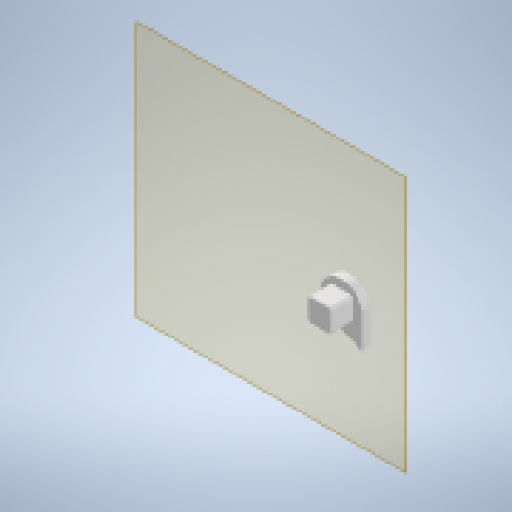
# Autodesk Inventor part: Arm
Saved by Autodesk Inventor 2025.2 (Build 292293000, 293)
## iProperties
Created: 2025-02-05
Part Number: Arm
Material: Generic
Document SubType Name: Modeling
Designer: andre
Density: 1 g/cm^3
Appearance: Default
Author: andre
Autodesk Inventor part; units mm, degrees
ref_plane "YZ Plane" through (0, 0, 0) normal (1, 0, 0) x (0, 1, 0)
ref_plane "XZ Plane" through (0, 0, 0) normal (0, 1, 0) x (-1, 0, 0)
ref_plane "XY Plane" through (0, 0, 0) normal (0, 0, 1) x (1, 0, 0)
ref_plane "Work Plane1" through (0, 0, 0) normal (0, 0, 1) x (1, 0, 0)
sketch "Sketch1" plane through (0, 0, 0) normal (0, 0, 1) x (1, 0, 0)
  line L0 (57, -9.5) -> (57, -71.5) projected
  line L1 (71, -71.5) -> (71, -9.5) projected
  line L2 (71, -40.5) -> (57, -40.5) construction
  circle A0 centre (64, -40.5) radius 7 construction
  circle A1 centre (64, -40.5) radius 6.6
  line L3 (70.6, -40.5) -> (70.6, -50.5)
  line L4 (70.6, -50.5) -> (61.4052, -46.5685)
  point P0 (0, 0)
  dimension "d0" = 0.4
  dimension "d1" = 10
  constraints: 6 end point, 3 midpoint, 2 point on circle, 2 tangent, 1 centre point, 1 horizontal alignment, 1 perpendicular, 1 point on line, 2 other
  measures "d1" distance of L3.start L3.end
extrude "Extrusion1" add sketch "Sketch1" along normal blind 2.7
sketch "Sketch2" plane through (0, 0, 2.7) normal (0, 0, 1) x (1, 0, 0)
  line L0 (61.4052, -46.5685) -> (70.6, -50.5) projected
  line L1 (70.6, -50.5) -> (70.6, -40.5) projected
  arc A0 (70.6, -40.5) -> (61.4052, -46.5685) centre (64, -40.5) ccw projected
  line L2 (58.5, -71.5) -> (58.5, -11) construction
  line L3 (69.5, -11) -> (69.5, -71.5) construction
  circle A1 centre (64, -40.5) radius 5.5 construction
  line L4 (60.2523, -36.7523) -> (67.7477, -36.7523)
  line L5 (67.7477, -36.7523) -> (67.7477, -44.2477)
  line L6 (67.7477, -44.2477) -> (60.2523, -44.2477)
  line L7 (60.2523, -44.2477) -> (60.2523, -36.7523)
  line L8 (60.0396, -36.6836) -> (67.9604, -44.3164) construction
  line L9 (67.7477, -36.7523) -> (60.2523, -44.2477) construction
  circle A2 centre (64, -40.5) radius 5.3
  point P0 (0, 0)
  dimension "d11" = 7.4953
  dimension "d12" = 7.4953
  dimension "d14" = 0.2
  constraints: 12 end point, 2 centre point, 2 midpoint, 2 parallel, 2 point on circle, 1 coincident, 1 horizontal, 1 other
  measures "d11" distance of L5.end L4.end
  measures "d12" distance of L5.end L6.end
  measures "d14" radial gap between concentric circles of A1 A2
extrude "Extrusion2" add sketch "Sketch2" along normal blind 7 contours L4 L5 L6 L7
fillet "Fillet1" radius 1 4 edges at (60.2523, -44.2477, 6.2) (60.2523, -36.7523, 6.2) (67.7477, -36.7523, 6.2) (67.7477, -44.2477, 6.2)
fillet "Fillet2" radius 0.5 8 edges at (67.4548, -43.9548, 9.7) (67.7477, -40.5, 9.7) (67.4548, -37.0452, 9.7) (64, -36.7523, 9.7) (60.5452, -37.0452, 9.7) (60.2523, -40.5, 9.7) (60.5452, -43.9548, 9.7) (64, -44.2477, 9.7)
equation "\"d12\" = d11"
body "Solid1"
